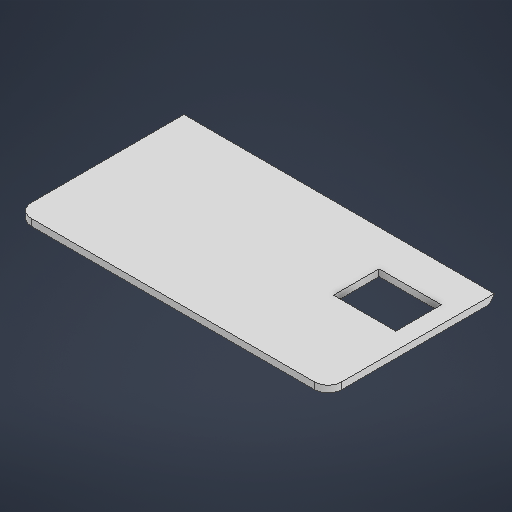
# Autodesk Inventor part: 前舵机位置控制
Saved by Autodesk Inventor 2025 (Build 290162000, 162)
## iProperties
Created: 2025-12-02
Part Number: 前舵机位置控制
Material: 常规
Document SubType Name: Modeling
Designer: HZD
Density: 1 g/cm^3
Appearance: 默认
Author: HZD
Autodesk Inventor part; units mm, degrees
ref_plane "YZ Plane" through (0, 0, 0) normal (1, 0, 0) x (0, 1, 0)
ref_plane "XZ Plane" through (0, 0, 0) normal (0, 1, 0) x (-1, 0, 0)
ref_plane "XY Plane" through (0, 0, 0) normal (0, 0, 1) x (1, 0, 0)
sketch "草图2" plane through (0, 0, 0) normal (0, 1, 0) x (-1, 0, 0)
  line L0 (-73.613, -25.5176) -> (7.387, -25.5176) projected
  line L1 (-73.613, -25.5176) -> (-73.613, 14.4824) projected
  line L2 (7.387, 14.4824) -> (-73.613, 14.4824) projected
  line L3 (7.387, -25.5176) -> (7.387, 14.4824) projected
  point P0 (0, 0)
extrude "拉伸1" add sketch "草图2" along normal blind 3
sketch "草图3" plane through (-7.387, 0, -25.5176) normal (-1, 0, 0) x (0, 0, 1)
  line L0 (0, 0) -> (40, 0) projected
  line L1 (0, 0) -> (-3, 0)
  line L2 (-3, 0) -> (-3, 26)
  line L3 (-3, 26) -> (0, 26)
  line L4 (0, 26) -> (0, 0)
  point P0 (25.5176, 0)
  dimension "d2" = 3
  dimension "d3" = 26
  constraints: 8 end point, 2 parallel, 1 horizontal, 1 perpendicular
  measures "d2" distance of L2.end L3.end
  measures "d3" distance between parallel lines of L1 L3
extrude "拉伸2" add sketch "草图3" against normal up to surface (81 mm away)
fillet "圆角1" radius 6.5 2 edges at (33.113, 3, -25.5176) (33.113, 0, -28.5176)
sketch "草图4" plane through (73.613, 26, -28.5176) normal (0, 0, -1) x (-1, 0, 0)
  line L0 (3, -1.1) -> (78, -1.1) projected
  line L1 (3, -76.1) -> (3, -1.1) projected
  line L2 (78, -76.1) -> (3, -76.1) projected
  line L3 (78, -1.1) -> (78, -76.1) projected
  line L4 (81, -79.1) -> (0, -79.1)
  line L5 (0, -79.1) -> (0, 1.9)
  line L6 (0, 1.9) -> (81, 1.9)
  line L7 (81, 1.9) -> (81, -79.1)
  line L8 (81, -8.1) -> (0, -8.1)
  line L9 (71, 1.9) -> (71, -79.1)
  line L10 (37.5, -29.6254) -> (37.5, -58.9595)
  line L11 (4, 1.9) -> (4, -79.1)
  point P0 (73.613, -26)
  point P1 (3, -8.1)
  point P2 (78, -8.1)
  dimension "d8" = 3
  dimension "d9" = 10
  dimension "d10" = 10
  constraints: 16 end point, 4 point on line, 2 perpendicular, 2 symmetric about line, 1 vertical, 3 other
  measures "d8" distance between parallel lines of L3 L7
  measures "d9" distance between parallel lines of L6 L8
  measures "d10" distance between parallel lines of L7 L9
extrude "拉伸3" add sketch "草图4" along normal blind 2 contours L1 L8 L5 L6 L11 L0 | L11 L6 L9 L0 | L9 L6 L7 L8 L3 L0
sketch "草图5" plane through (73.613, 26, -28.5176) normal (0, 0, 1) x (1, 0, 0)
  line L0 (0, 1.9) -> (0, 0) projected
  line L1 (-81, 1.9) -> (0, 1.9) projected
  line L2 (-81, 0) -> (-81, 1.9) projected
  line L3 (-81, 0) -> (0, 0) projected
  point P0 (-73.613, -26)
extrude "拉伸4" add sketch "草图5" along normal up to surface (3 mm away)
sketch "草图6" plane through (0, 0, 0) normal (0, -1, 0) x (1, 0, 0)
  point P0 (0, 0)
sketch "草图7" plane through (0, 0, 0) normal (0, -1, 0) x (1, 0, 0)
  line L0 (-4.387, -23.5176) -> (-7.387, -23.5176) projected
  line L1 (-4.387, -23.5176) -> (-4.387, 10.4824) projected
  line L2 (-4.387, 10.4824) -> (70.613, 10.4824) projected
  line L3 (70.613, 10.4824) -> (70.613, -23.5176) projected
  line L4 (73.613, -23.5176) -> (70.613, -23.5176) projected
  line L5 (73.613, -23.5176) -> (73.613, 14.4824) projected
  line L6 (-7.387, 14.4824) -> (73.613, 14.4824) projected
  line L7 (-7.387, -23.5176) -> (-7.387, 14.4824) projected
  circle A0 centre (-1.887, 7.4824) radius 1
  circle A1 centre (-1.887, 3.7324) radius 1
  circle A2 centre (-1.887, -0.0176) radius 1
  line L8 (-0.012, 10.0781) -> (-0.012, 2.7913)
  circle A3 centre (1.863, 7.4824) radius 1
  circle A4 centre (1.863, 3.7324) radius 1
  circle A5 centre (1.863, -0.0176) radius 1
  point P0 (0, 0)
  dimension "d16" = 3.75
  dimension "d17" = 3.75
  dimension "d18" = 2
  dimension "d19" = 2
  dimension "d20" = 2
  dimension "d22" = 1.875
  dimension "d32" = 3
  dimension "d78" = 2.5
  constraints: 6 centre point, 3 symmetric about line, 2 end point, 2 vertical alignment, 1 vertical, 3 other
  measures "d16" distance of A1.centre A0.centre
  measures "d17" distance of A1.centre A2.centre
  measures "d18" diameter of A2
  measures "d19" diameter of A1
  measures "d20" diameter of A0
  measures "d22" distance from line of A1.centre L8
  measures "d32" distance from line of L2 A3.centre
  measures "d78" distance from line of A0.centre L1
extrude "拉伸5" cut sketch "草图7" against normal blind 2 contours A0 | A1 | A2 | A3 | A4 | A5
fillet "圆角3" radius 0.3 6 edges at (-2.887, 2, 7.4824) (0.863, 2, 7.4824) (0.863, 2, 3.7324) (-2.887, 2, 3.7324) (0.863, 2, -0.0176) (-2.887, 2, -0.0176)
chamfer "倒角1" distance 0.5 angle 45 6 edges at (0.863, 0, 7.4824) (0.863, 0, 3.7324) (0.863, 0, -0.0176) (-2.887, 0, 3.7324) (-2.887, 0, 7.4824) (-2.887, 0, -0.0176)
pattern_linear "矩形阵列1" count 8 spacing 9 along (1, 0, 0) of "拉伸5", "圆角3", "倒角1"
pattern_linear "矩形阵列2" count 2 spacing 15 along (0, 0, -1) of "拉伸5", "圆角3", "倒角1", "矩形阵列1"
sketch "草图8" plane through (-7.387, 0, 14.4824) normal (-1, 0, 0) x (0, 0, 1)
  line L0 (-34.4531, 29.25) -> (-48.8428, 29.25)
  line L1 (-48.8428, 29.25) -> (-48.8428, 9.5)
  line L2 (-48.8428, 9.5) -> (-34.4531, 9.5)
  line L3 (-34.4531, 9.5) -> (-34.4531, 29.25)
  point P0 (-14.4824, 0)
  point P1 (-40, 9.5)
  constraints: 8 end point, 2 parallel, 1 horizontal, 1 perpendicular, 1 point on line
extrude "拉伸6" cut sketch "草图8" against normal blind 138.5
move faces "移动1" translate (34, 0, 0) faces at (73.613, 1, -8.8509)
sketch "草图10" plane through (0, 3, 0) normal (0, 1, 0) x (1, 0, 0)
  line L0 (70.0223, 10.5176) -> (109.2642, 10.5176)
  line L1 (109.2642, 10.5176) -> (109.2642, 51.6366)
  line L2 (109.2642, 51.6366) -> (70.0223, 51.6366)
  line L3 (70.0223, 51.6366) -> (70.0223, 10.5176)
  line L4 (70.0223, 58.5176) -> (70.0223, 28.5176)
  point P0 (0, 0)
  constraints: 10 end point, 2 parallel, 1 collinear, 1 horizontal, 1 perpendicular, 1 vertical, 2 other
extrude "拉伸8" cut sketch "草图10" along normal blind 55.75
delete faces "删除1" heal yes whole lump no faces at (44.2192, 5.0789, -23.7824)
fillet "圆角6" radius 2 2 edges at (-7.387, 0, -3.7676) (-7.387, 0.7991, -25.1401)
sketch "草图18" plane through (107.613, 0, 14.4824) normal (1, 0, 0) x (0, 0, -1)
  arc A0 (36.5, 0) -> (41.9772, 3) centre (36.5, 6.5) ccw projected
  line L0 (36.5, 0) -> (41.9772, 0)
  line L1 (41.9772, 0) -> (41.9772, 3)
  line L2 (41.9772, 3) -> (36.5, 3)
  line L3 (36.5, 3) -> (36.5, 0)
  point P0 (14.4824, 0)
  constraints: 8 end point, 2 parallel, 1 horizontal, 1 perpendicular
delete faces "删除3" heal yes whole lump no faces at (-7.2982, 1.4105, 2.3158) (-6.321, 0.578, -24.0729)
extrude "拉伸15" add sketch "草图18" against normal up to surface (115 mm away) contours A0 L1 L0
sketch "草图19" plane through (-7.387, 3, 14.4824) normal (0, 1, 0) x (1, 0, 0)
  arc A0 (111.7381, -34.2953) -> (117.7381, -28.2953) centre (111.7381, -28.2953) ccw
  line L0 (-20.2551, 42.7047) -> (117.7381, 42.7047)
  line L1 (117.7381, 42.7047) -> (117.7381, -34.2953)
  line L2 (117.7381, -34.2953) -> (-20.2551, -34.2953)
  line L3 (-20.2551, -34.2953) -> (-20.2551, 42.7047)
  line L4 (0, 41.9772) -> (115, 41.9772) projected
  line L5 (0, 41.9772) -> (0, 0) projected
  line L6 (0, 0) -> (115, 0) projected
  line L7 (115, 0) -> (115, 41.9772) projected
  line L8 (0, 41.9772) -> (0, 0) projected
  line L9 (115, 41.9772) -> (0, 41.9772) projected
  line L10 (115, 0) -> (115, 41.9772) projected
  line L11 (0, 0) -> (115, 0) projected
  circle A1 centre (5.5, 14.5) radius 1.5 projected
  circle A2 centre (5.5, 10.75) radius 1.5 projected
  circle A3 centre (5.5, 7) radius 1.5 projected
  circle A4 centre (9.25, 7) radius 1.5 projected
  circle A5 centre (9.25, 10.75) radius 1.5 projected
  circle A6 centre (9.25, 14.5) radius 1.5 projected
  circle A7 centre (14.5, 14.5) radius 1.5 projected
  circle A8 centre (14.5, 10.75) radius 1.5 projected
  circle A9 centre (14.5, 7) radius 1.5 projected
  circle A10 centre (18.25, 7) radius 1.5 projected
  circle A11 centre (18.25, 10.75) radius 1.5 projected
  circle A12 centre (18.25, 14.5) radius 1.5 projected
  circle A13 centre (23.5, 14.5) radius 1.5 projected
  circle A14 centre (23.5, 10.75) radius 1.5 projected
  circle A15 centre (23.5, 7) radius 1.5 projected
  circle A16 centre (27.25, 7) radius 1.5 projected
  circle A17 centre (27.25, 10.75) radius 1.5 projected
  circle A18 centre (27.25, 14.5) radius 1.5 projected
  circle A19 centre (32.5, 14.5) radius 1.5 projected
  circle A20 centre (32.5, 10.75) radius 1.5 projected
  circle A21 centre (32.5, 7) radius 1.5 projected
  circle A22 centre (36.25, 7) radius 1.5 projected
  circle A23 centre (36.25, 10.75) radius 1.5 projected
  circle A24 centre (36.25, 14.5) radius 1.5 projected
  circle A25 centre (41.5, 14.5) radius 1.5 projected
  circle A26 centre (41.5, 10.75) radius 1.5 projected
  circle A27 centre (41.5, 7) radius 1.5 projected
  circle A28 centre (45.25, 7) radius 1.5 projected
  circle A29 centre (45.25, 10.75) radius 1.5 projected
  circle A30 centre (45.25, 14.5) radius 1.5 projected
  circle A31 centre (50.5, 14.5) radius 1.5 projected
  circle A32 centre (50.5, 10.75) radius 1.5 projected
  circle A33 centre (50.5, 7) radius 1.5 projected
  circle A34 centre (54.25, 7) radius 1.5 projected
  circle A35 centre (54.25, 10.75) radius 1.5 projected
  circle A36 centre (54.25, 14.5) radius 1.5 projected
  circle A37 centre (59.5, 14.5) radius 1.5 projected
  circle A38 centre (59.5, 10.75) radius 1.5 projected
  circle A39 centre (59.5, 7) radius 1.5 projected
  circle A40 centre (63.25, 7) radius 1.5 projected
  circle A41 centre (63.25, 10.75) radius 1.5 projected
  circle A42 centre (63.25, 14.5) radius 1.5 projected
  circle A43 centre (68.5, 14.5) radius 1.5 projected
  circle A44 centre (68.5, 10.75) radius 1.5 projected
  circle A45 centre (68.5, 7) radius 1.5 projected
  circle A46 centre (72.25, 7) radius 1.5 projected
  circle A47 centre (72.25, 10.75) radius 1.5 projected
  circle A48 centre (72.25, 14.5) radius 1.5 projected
  circle A49 centre (5.5, 29.5) radius 1.5 projected
  circle A50 centre (5.5, 25.75) radius 1.5 projected
  circle A51 centre (5.5, 22) radius 1.5 projected
  circle A52 centre (9.25, 22) radius 1.5 projected
  circle A53 centre (9.25, 25.75) radius 1.5 projected
  circle A54 centre (9.25, 29.5) radius 1.5 projected
  circle A55 centre (14.5, 29.5) radius 1.5 projected
  circle A56 centre (14.5, 25.75) radius 1.5 projected
  circle A57 centre (14.5, 22) radius 1.5 projected
  circle A58 centre (18.25, 22) radius 1.5 projected
  circle A59 centre (18.25, 25.75) radius 1.5 projected
  circle A60 centre (18.25, 29.5) radius 1.5 projected
  circle A61 centre (23.5, 29.5) radius 1.5 projected
  circle A62 centre (23.5, 25.75) radius 1.5 projected
  circle A63 centre (23.5, 22) radius 1.5 projected
  circle A64 centre (27.25, 22) radius 1.5 projected
  circle A65 centre (27.25, 25.75) radius 1.5 projected
  circle A66 centre (27.25, 29.5) radius 1.5 projected
  circle A67 centre (32.5, 29.5) radius 1.5 projected
  circle A68 centre (32.5, 25.75) radius 1.5 projected
  circle A69 centre (32.5, 22) radius 1.5 projected
  circle A70 centre (36.25, 22) radius 1.5 projected
  circle A71 centre (36.25, 25.75) radius 1.5 projected
  circle A72 centre (36.25, 29.5) radius 1.5 projected
  circle A73 centre (41.5, 29.5) radius 1.5 projected
  circle A74 centre (41.5, 25.75) radius 1.5 projected
  circle A75 centre (41.5, 22) radius 1.5 projected
  circle A76 centre (45.25, 22) radius 1.5 projected
  circle A77 centre (45.25, 25.75) radius 1.5 projected
  circle A78 centre (45.25, 29.5) radius 1.5 projected
  circle A79 centre (50.5, 29.5) radius 1.5 projected
  circle A80 centre (50.5, 25.75) radius 1.5 projected
  circle A81 centre (50.5, 22) radius 1.5 projected
  circle A82 centre (54.25, 22) radius 1.5 projected
  circle A83 centre (54.25, 25.75) radius 1.5 projected
  circle A84 centre (54.25, 29.5) radius 1.5 projected
  circle A85 centre (59.5, 29.5) radius 1.5 projected
  circle A86 centre (59.5, 25.75) radius 1.5 projected
  circle A87 centre (59.5, 22) radius 1.5 projected
  circle A88 centre (63.25, 22) radius 1.5 projected
  circle A89 centre (63.25, 25.75) radius 1.5 projected
  circle A90 centre (63.25, 29.5) radius 1.5 projected
  circle A91 centre (68.5, 29.5) radius 1.5 projected
  circle A92 centre (68.5, 25.75) radius 1.5 projected
  circle A93 centre (68.5, 22) radius 1.5 projected
  circle A94 centre (72.25, 22) radius 1.5 projected
  circle A95 centre (72.25, 25.75) radius 1.5 projected
  circle A96 centre (72.25, 29.5) radius 1.5 projected
  point P0 (111.7381, -34.2953)
  point P1 (117.7381, -28.2953)
  constraints: 8 end point, 2 parallel, 2 point on circle, 1 centre point, 1 horizontal, 1 perpendicular, 5 other
extrude "拉伸16" add sketch "草图19" against normal blind 3 contours L2 L3 L0 L1 A0
fillet "圆角7" radius 6 1 edges at (-27.6421, 1.5, 48.7778)
sketch "草图20" plane through (110.3511, 3, 42.7778) normal (1, 0, 0) x (0, 0, -1)
  line L0 (66.3497, -2.1735) -> (69.0116, 1.5)
  spline S0 degree 3 poles (66.3497, -2.1735) (66.2851, -2.2627) (66.2134, -2.346) (65.9612, -2.5956) (65.7378, -2.7479) (65.2475, -2.9501) (64.9805, -3) (64.7302, -3) knots 0 0 0 0 0.178498 0.178498 0.589249 0.589249 1 1 1 1
  line L1 (26, -3) -> (66, -3)
  line L2 (0, 0) -> (71, 0)
  line L3 (71, -3) -> (0, -3)
  line L4 (71, 0) -> (71, -3)
  line L5 (0, 0) -> (71, 0)
  line L6 (0, 0) -> (0, -3)
  point P0 (42.7778, -3)
  point P1 (67.9247, 0)
  point P2 (66, -3)
  constraints: 4 end point, 1 horizontal, 8 other
extrude "拉伸17" cut sketch "草图20" against normal blind 182.75 contours L0 L2 L4 L3 L1 S0
sketch "草图21" plane through (-21.6421, 3, 48.7778) normal (0, 1, 0) x (1, 0, 0)
  line L0 (124.4663, 57.9002) -> (96.7663, 57.8614)
  line L1 (124.4663, 57.9002) -> (124.4947, 37.6402)
  line L2 (124.4947, 37.6402) -> (96.7947, 37.6014)
  line L3 (96.7947, 37.6014) -> (96.7663, 57.8614)
  point P0 (21.6421, 48.7778)
  constraints: 8 end point, 8 other
extrude "拉伸18" cut sketch "草图21" against normal blind 10
sketch "草图23" plane through (-21.6421, 0, 48.7778) normal (0, -1, 0) x (1, 0, 0)
  line L0 (-4.0068, -26) -> (-4.0068, -16)
  line L1 (-4.0068, -16) -> (0.9932, -16)
  line L2 (0.9932, -16) -> (0.9932, -26)
  line L3 (0.9932, -26) -> (-4.0068, -26)
  line L4 (0.9932, -49) -> (-4.0068, -49)
  line L5 (-4.0068, -49) -> (-4.0068, -59)
  line L6 (0.9932, -59) -> (0.9932, -49)
  line L7 (-4.0068, -59) -> (0.9932, -59)
  line L8 (129.9865, -16) -> (124.9865, -16)
  line L9 (129.9865, -26) -> (129.9865, -16)
  line L10 (124.9865, -16) -> (124.9865, -26)
  line L11 (124.9865, -26) -> (129.9865, -26)
  point P0 (21.6421, -48.7778)
  constraints: 24 end point, 6 horizontal, 6 vertical, 12 other
extrude "拉伸19" cut sketch "草图23" against normal blind 1.5
